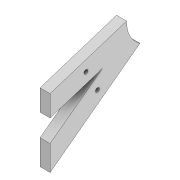
# Autodesk Inventor part: Horizontal_bar_reinforcement_V2
Saved by Autodesk Inventor 2022 (Build 260153000, 153)
## iProperties
Created: 2022-08-23
Part Number: Horizontal_bar_reinforcement_V2
Material: Generic
Document SubType Name: Modeling
Designer: dell
Density: 1 g/cm^3
Appearance: Default
Mass: 25.8229 g
Surface Area: 170.293 cm^2
Volume: 25.8229 cm^3
Author: dell
Autodesk Inventor part; units mm, degrees
ref_plane "YZ Plane" through (0, 0, 0) normal (1, 0, 0) x (0, 1, 0)
ref_plane "XZ Plane" through (0, 0, 0) normal (0, 1, 0) x (-1, 0, 0)
ref_plane "XY Plane" through (0, 0, 0) normal (0, 0, 1) x (1, 0, 0)
sketch "Sketch1" plane through (0, 0, 0) normal (1, 0, 0) x (0, 1, 0)
  circle A0 centre (0, -124) radius 1.95
  circle A1 centre (0, 124) radius 1.95
  circle A2 centre (-19, -65) radius 1.5
  circle A3 centre (-19, 65) radius 1.5
  line L0 (0, 124) -> (-19, 65) construction
  line L1 (4.7593, 122.4673) -> (-14.2407, 63.4673)
  line L2 (-23.7593, 66.5327) -> (-4.7593, 125.5327)
  arc A4 (4.7593, 122.4673) -> (-4.7593, 125.5327) centre (0, 124) ccw
  arc A5 (-23.7593, 66.5327) -> (-14.2407, 63.4673) centre (-19, 65) ccw
  line L3 (-19, 65) -> (-19, -65) construction
  line L4 (-24, 65) -> (-24, -65)
  line L5 (-14, -65) -> (-14, 65)
  arc A6 (-14, 65) -> (-24, 65) centre (-19, 65) ccw
  arc A7 (-24, -65) -> (-14, -65) centre (-19, -65) ccw
  line L6 (-19, -65) -> (0, -124) construction
  line L7 (-23.7593, -66.5327) -> (-4.7593, -125.5327)
  line L8 (4.7593, -122.4673) -> (-14.2407, -63.4673)
  arc A8 (-14.2407, -63.4673) -> (-23.7593, -66.5327) centre (-19, -65) ccw
  arc A9 (-4.7593, -125.5327) -> (4.7593, -122.4673) centre (0, -124) ccw
  circle A10 centre (-44, 65) radius 1.5
  circle A11 centre (-44, -65) radius 1.5
  line L9 (-19, 65) -> (-44, 65) construction
  line L10 (-19, 67) -> (-44, 67)
  line L11 (-44, 63) -> (-19, 63)
  arc A12 (-19, 63) -> (-19, 67) centre (-19, 65) ccw
  arc A13 (-44, 67) -> (-44, 63) centre (-44, 65) ccw
  line L12 (-19, -65) -> (-44, -65) construction
  line L13 (-19, -63) -> (-44, -63)
  line L14 (-44, -67) -> (-19, -67)
  arc A14 (-19, -67) -> (-19, -63) centre (-19, -65) ccw
  arc A15 (-44, -63) -> (-44, -67) centre (-44, -65) ccw
  line L15 (0, 124) -> (-44, 65) construction
  line L16 (-4.0081, 126.9891) -> (-48.0081, 67.9891)
  line L17 (-39.9919, 62.0109) -> (4.0081, 121.0109)
  arc A16 (4.0081, 121.0109) -> (-4.0081, 126.9891) centre (0, 124) ccw
  arc A17 (-48.0081, 67.9891) -> (-39.9919, 62.0109) centre (-44, 65) ccw
  line L18 (-44, -65) -> (0, -124) construction
  line L19 (-48.0081, -67.9891) -> (-4.0081, -126.9891)
  line L20 (4.0081, -121.0109) -> (-39.9919, -62.0109)
  arc A18 (-39.9919, -62.0109) -> (-48.0081, -67.9891) centre (-44, -65) ccw
  arc A19 (-4.0081, -126.9891) -> (4.0081, -121.0109) centre (0, -124) ccw
  line L21 (-44, 65) -> (-44, -65) construction
  line L22 (-46.5, 65) -> (-46.5, -65)
  line L23 (-41.5, -65) -> (-41.5, 65)
  arc A20 (-41.5, 65) -> (-46.5, 65) centre (-44, 65) ccw
  arc A21 (-46.5, -65) -> (-41.5, -65) centre (-44, -65) ccw
  line L24 (-44, 65) -> (-19, 0) construction
  line L25 (-45.4, 64.4615) -> (-20.4, -0.5385)
  line L26 (-17.6, 0.5385) -> (-42.6, 65.5385)
  arc A22 (-42.6, 65.5385) -> (-45.4, 64.4615) centre (-44, 65) ccw
  arc A23 (-20.4, -0.5385) -> (-17.6, 0.5385) centre (-19, 0) ccw
  line L27 (-44, -65) -> (-19, 0) construction
  line L28 (-42.6, -65.5385) -> (-17.6, -0.5385)
  line L29 (-20.4, 0.5385) -> (-45.4, -64.4615)
  arc A24 (-45.4, -64.4615) -> (-42.6, -65.5385) centre (-44, -65) ccw
  arc A25 (-17.6, -0.5385) -> (-20.4, 0.5385) centre (-19, 0) ccw
  line L30 (-19, 0) -> (-44, 0) construction
  line L31 (-19, 1.5) -> (-44, 1.5)
  line L32 (-44, -1.5) -> (-19, -1.5)
  arc A26 (-19, -1.5) -> (-19, 1.5) centre (-19, 0) ccw
  arc A27 (-44, 1.5) -> (-44, -1.5) centre (-44, 0) ccw
  circle A28 centre (-19, -10) radius 1.5
  circle A29 centre (-19, -35) radius 1.5
  circle A30 centre (-19, 10) radius 1.5
  circle A31 centre (-19, 35) radius 1.5
  circle A32 centre (0, -124) radius 12.5
  circle A33 centre (0, 124) radius 12.5
  circle A34 centre (-22, 94.5) radius 1
  circle A35 centre (-22, -94.5) radius 1
  circle A36 centre (-11.3392, 88.7888) radius 1
  circle A37 centre (-11.3392, -88.7888) radius 1
  circle A38 centre (-19, 0) radius 1
  point P0 (0, 0)
  point P1 (-9.5, 94.5)
  point P2 (-9.5, -94.5)
  point P3 (-14, -64.2148)
  point P4 (-14, 64.2148)
  point P5 (-24, 65)
  point P6 (-31.5, 65)
  point P7 (-31.5, -65)
  point P8 (-44, 0)
  point P9 (-31.5, 32.5)
  point P10 (-31.5, -32.5)
  point P11 (-41.5, 54.3215)
  point P12 (-24, 8.8215)
  point P13 (-24, 17.1785)
  point P14 (-41.6236, 63)
  point P15 (-24, 63)
  point P16 (-23.6088, 67)
  point P17 (-36.2712, 67)
  point P18 (-13.9854, 96.8832)
  point P19 (-6.8749, 118.9633)
  point P20 (-43.3898, 70)
  point P21 (-46.5, -65)
  point P22 (-43.3898, -70)
  point P23 (-6.8749, -118.9633)
  point P24 (-13.9854, -96.8832)
  point P25 (-36.2712, -67)
  point P26 (-23.6088, -67)
  point P27 (-24, -63)
  point P28 (-41.6236, -63)
  point P29 (-24, -17.1785)
  point P30 (-24, -8.8215)
  point P31 (-41.5, -54.3215)
  point P32 (-31.5, 0)
  point P33 (-41.5, -1.5)
  point P34 (-24, -1.5)
  point P35 (-24, 1.5)
  point P36 (-41.5, 1.5)
  point P37 (-46.5, 60.6699)
  point P38 (-46.5, -60.6699)
  point P39 (-4.0081, -126.9891)
  point P40 (-41.5, 63)
  point P41 (-23.5826, 67)
  point P42 (-41.5, -63)
  point P43 (-41.5, -62.6785)
  point P44 (-41.5, 62.6785)
  point P45 (-10.8571, -117.8053)
  point P46 (1.2475, -111.5624)
  point P47 (-10.8571, 117.8053)
  point P48 (1.2475, 111.5624)
  point P49 (-40.8878, -61.0867)
  point P50 (-41.5, 60.6699)
  dimension "d2" = 3.9
  dimension "d4" = 3.9
  dimension "d25" = 3
  dimension "d28" = 3
  dimension "d43" = 59
  dimension "d44" = 65
  dimension "d45" = 65
  dimension "d47" = 59
  dimension "d48" = 10
  dimension "d49" = 10
  dimension "d50" = 10
  dimension "d52" = 14
  dimension "d53" = 3
  dimension "d54" = 3
  dimension "d55" = 4
  dimension "d56" = 4
  dimension "d57" = 25
  dimension "d58" = 25
  dimension "d59" = 10
  dimension "d60" = 10
  dimension "d61" = 5
  dimension "d62" = 3
  dimension "d63" = 3
  dimension "d64" = 3
  dimension "d65" = 3
  dimension "d66" = 3
  dimension "d67" = 10
  dimension "d68" = 25
  dimension "d69" = 3
  dimension "d70" = 3
  dimension "d71" = 10
  dimension "d72" = 25
  dimension "d73" = 25
  dimension "d74" = 25
  dimension "d76" = 2
  dimension "d78" = 2
  dimension "d79" = 2
  dimension "d80" = 2
  dimension "d81" = 6
  dimension "d82" = 6
  dimension "d83" = 2
  constraints: 88 end point, 44 point on circle, 44 tangent, 39 centre point, 11 midpoint, 11 parallel, 6 coincident, 6 point on line, 3 vertical alignment, 2 horizontal alignment, 1 concentric, 1 horizontal, 1 perpendicular, 1 vertical
  measures "d2" diameter of A0
  measures "d4" diameter of A1
  measures "d25" diameter of A2
  measures "d28" diameter of A3
  measures "d43" vertical distance of L0.start L0.end
  measures "d44" vertical distance of point (0, 0) L0.end
  measures "d45" vertical distance of point (0, 0) L3.end
  measures "d47" vertical distance of L3.end L6.end
  measures "d48" distance between parallel lines of L1 L2
  measures "d49" distance between parallel lines of L4 L5
  measures "d50" distance between parallel lines of L7 L8
  measures "d52" distance from line of point (0, 0) L5
  measures "d53" diameter of A10
  measures "d54" diameter of A11
  measures "d55" diameter of A13
  measures "d56" diameter of A15
  measures "d57" distance of L0.end L9.end
  measures "d58" distance of L3.end L12.end
  measures "d59" diameter of A17
  measures "d60" diameter of A19
  measures "d61" diameter of A21
  measures "d62" diameter of A23
  measures "d63" diameter of A25
  measures "d64" diameter of A27
  measures "d65" diameter of A28
  measures "d66" diameter of A29
  measures "d67" distance of L24.end A28.centre
  measures "d68" distance of A28.centre A29.centre
  measures "d69" diameter of A30
  measures "d70" diameter of A31
  measures "d71" distance of L24.end A30.centre
  measures "d72" distance of A30.centre A31.centre
  measures "d73" diameter of A32
  measures "d74" diameter of A33
  measures "d76" diameter of A34
  measures "d78" diameter of A35
  measures "d79" diameter of A36
  measures "d80" diameter of A37
  measures "d81" distance of point (-9.5, -94.5) A37.centre
  measures "d82" distance of A36.centre point (-9.5, 94.5)
  measures "d83" diameter of A38
extrude "Extrusion1" add sketch "Sketch1" along normal blind 5 contours A4 L16 A33 L1 | A16 L17 A33 L2 A4 | L1 A33 L17 A16 | L1 L5 A6 L10 L2 L17 A33 | A4 L2 A33 L16 | L5 L8 A8 L13 L4 L28 A23 L26 L11 A5 L1 | L1 A5 L11 A12 L10 A6 L5 | L17 L2 A33 | A33 L2 L17 L10 A20 L22 A17 L16 | L8 A32 L20 L7 L14 A7 L5 | L5 A7 L14 A14 L13 A8 L8 | L11 L4 A5 | A5 A6 L10 A12 L11 | A32 L19 A9 L8 | L8 A19 L20 A32 | A6 L2 L10 | L2 A5 L4 L11 L17 L10 | L17 L11 L23 A20 L10 | L22 A20 L10 A13 L25 A17 | A17 L25 L23 L31 A27 L32 L29 A18 L22 | L14 L7 A7 | A7 A8 L13 A14 L14 | A9 L7 A32 L20 A19 | A32 L7 L20 | A8 L4 L13 | A20 L23 L11 L26 A10 L25 A13 L10 | L25 A13 L11 L26 L23 A17 | A17 L23 L25 | L22 A21 L14 L20 L7 A32 L19 A18 | A18 L29 A15 L14 A21 L22 | L26 A25 L31 L25 L4 | L4 L25 L23 A17 L26 | L7 L14 L20 L13 L4 A7 | L19 A32 L7 A9 | L23 L26 L11 | L23 L26 A17 | L25 A10 L26 L11 A13 | L29 L23 A18 | A18 L23 L28 L13 A15 L29 | L25 L31 L4 | A23 L25 L29 A25 | L14 A21 L23 L13 L20 | L28 A18 L23 L29 L4 | L4 L29 L32 A23 L28 | L31 L4 L32 L23 | L23 L32 A27 L31 | A18 L28 L23 | L29 A11 L28 L13 L23 A21 L14 A15 | A15 L13 L28 A11 L29 | L31 L25 L29 L32 L4 | L31 A25 L29 L25 | L4 L32 L29 | L25 A23 L32 L29
sketch "Sketch8" plane through (5, 0, 0) normal (1, 0, 0) x (0, 0, -1)
  line L0 (-54.3215, -41.5) -> (-1.5, -41.5) projected
  line L1 (-1.5, -41.5) -> (-1.5, -24) projected
  line L2 (-1.5, -24) -> (-8.8215, -24) projected
  line L3 (-8.8215, -24) -> (-54.3215, -41.5) projected
  line L4 (1.5, -24) -> (1.5, -41.5) projected
  line L5 (1.5, -41.5) -> (54.3215, -41.5) projected
  line L6 (54.3215, -41.5) -> (8.8215, -24) projected
  line L7 (8.8215, -24) -> (1.5, -24) projected
  line L8 (-67, -23.6088) -> (-96.8832, -13.9854) projected
  line L9 (-96.8832, -13.9854) -> (-67, -36.2712) projected
  line L10 (-67, -36.2712) -> (-67, -23.6088) projected
  line L11 (63, -24) -> (17.1785, -24) projected
  line L12 (17.1785, -24) -> (63, -41.6236) projected
  line L13 (63, -41.6236) -> (63, -24) projected
  circle A0 centre (-65, -44) radius 1.5 projected
  circle A1 centre (124, 0) radius 1.95 projected
  circle A2 centre (-124, 0) radius 1.95 projected
  circle A3 centre (-94.5, -22) radius 1 projected
  circle A4 centre (-35, -19) radius 1.5 projected
  circle A5 centre (-10, -19) radius 1.5 projected
  circle A6 centre (35, -19) radius 1.5 projected
  circle A7 centre (10, -19) radius 1.5 projected
  circle A8 centre (65, -19) radius 1.5 projected
  circle A9 centre (88.7888, -11.3392) radius 1 projected
  circle A10 centre (-65, -19) radius 1.5 projected
  circle A11 centre (-88.7888, -11.3392) radius 1 projected
  circle A12 centre (94.5, -22) radius 1 projected
  circle A13 centre (65, -44) radius 1.5 projected
  line L14 (67, -23.6088) -> (67, -36.2712) projected
  line L15 (67, -36.2712) -> (96.8832, -13.9854) projected
  line L16 (96.8832, -13.9854) -> (67, -23.6088) projected
  line L17 (-62.6785, -41.5) -> (-17.1785, -24) projected
  line L18 (-17.1785, -24) -> (-63, -24) projected
  line L19 (-63, -24) -> (-63, -41.5) projected
  line L20 (-63, -41.5) -> (-62.6785, -41.5) projected
  arc A14 (117.8053, -10.8571) -> (111.5624, 1.2475) centre (124, 0) ccw projected
  line L21 (117.8053, -10.8571) -> (67.9891, -48.0081) projected
  arc A15 (60.6699, -46.5) -> (67.9891, -48.0081) centre (65, -44) ccw projected
  line L22 (60.6699, -46.5) -> (-60.6699, -46.5) projected
  arc A16 (-67.9891, -48.0081) -> (-60.6699, -46.5) centre (-65, -44) ccw projected
  line L23 (-67.9891, -48.0081) -> (-117.8053, -10.8571) projected
  arc A17 (-111.5624, 1.2475) -> (-117.8053, -10.8571) centre (-124, 0) ccw projected
  line L24 (-111.5624, 1.2475) -> (-64.2148, -14) projected
  line L25 (-64.2148, -14) -> (64.2148, -14) projected
  line L26 (64.2148, -14) -> (111.5624, 1.2475) projected
  circle A18 centre (0, -19) radius 1 projected
  point P0 (0, 0)
sketch "Sketch9" plane through (5, 0, 0) normal (1, 0, 0) x (0, 0, -1)
  circle A0 centre (124, 0) radius 1.95 projected
  circle A1 centre (124, 0) radius 15
  line L0 (111.5624, 1.2475) -> (64.2148, -14) projected
  circle A2 centre (88.7888, -11.3392) radius 1 projected
  line L1 (67, -23.6088) -> (96.8832, -13.9854) projected
  line L2 (96.8832, -13.9854) -> (67, -36.2712) projected
  line L3 (67.9891, -48.0081) -> (117.8053, -10.8571) projected
  circle A3 centre (94.5, -22) radius 1 projected
  line L4 (71, -11.8149) -> (71, -45.7627)
  circle A4 centre (65, -19) radius 1.5 projected
  point P0 (0, 0)
  point P1 (71, -33.2881)
  point P2 (115.6524, -12.4626)
  point P3 (109.006, 0.4243)
  point P4 (71, -22.3207)
  dimension "d84" = 30
  dimension "d85" = 6
  constraints: 2 end point, 2 point on line, 1 centre point, 1 coincident, 1 vertical
  measures "d84" diameter of A1
  measures "d85" distance from line of A4.centre L4
extrude "Extrusion4" add sketch "Sketch9" along normal blind 5 contours A1 L3 L4 L2 L1 L0
sketch "Sketch10" plane through (5, 0, 0) normal (1, 0, 0) x (0, 0, -1)
  line L0 (-181.8877, 79.6872) -> (179.0889, 79.6872)
  line L1 (179.0889, 79.6872) -> (179.0889, -93.8152)
  line L2 (179.0889, -93.8152) -> (-181.8877, -93.8152)
  line L3 (-181.8877, -93.8152) -> (-181.8877, 79.6872)
  point P0 (0, 0)
  constraints: 8 end point, 2 parallel, 1 horizontal, 1 perpendicular
extrude "Extrusion5" cut sketch "Sketch10" against normal blind 10
body "Solid1"
